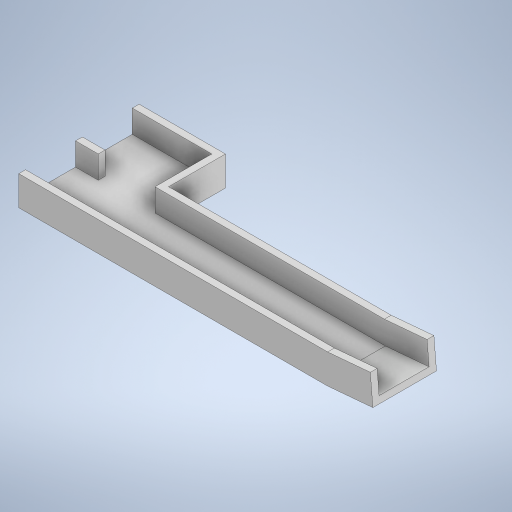
# Autodesk Inventor part: Trilho 5 min
Saved by Autodesk Inventor 2024 (Build 280153020, 153B)
## iProperties
Created: 2023-05-22
Part Number: Trilho 5 min
Material: Genérico
Document SubType Name: Modeling
Designer: jpjoa
Density: 1 g/cm^3
Appearance: Padrão
Author: jpjoa
Autodesk Inventor part; units mm, degrees
ref_plane "YZ Plane" through (0, 0, 0) normal (1, 0, 0) x (0, 1, 0)
ref_plane "XZ Plane" through (0, 0, 0) normal (0, 1, 0) x (-1, 0, 0)
sketch "Esboço1" plane through (0, 0, 0) normal (0, 1, 0) x (-1, 0, 0)
  line L0 (-133, -3) -> (0, -3)
  line L1 (0, -25) -> (-98, -25)
  line L2 (-133, 0) -> (-133, -28)
  line L3 (-133, -28) -> (-123, -28)
  line L4 (-95, -28) -> (0, -28)
  line L5 (0, -28) -> (0, 0)
  line L6 (0, 0) -> (-133, 0)
  line L7 (-95, -28) -> (-95, -53)
  line L8 (-95, -53) -> (-133, -53)
  line L9 (-133, -53) -> (-133, -50)
  line L10 (-133, -50) -> (-98, -50)
  line L11 (-98, -50) -> (-98, -25)
  arc A0 (-123, -50) -> (-98, -25) centre (-123, -25) ccw
  arc A1 (-123, -28) -> (-120, -25) centre (-123, -25) ccw
  line L12 (-133, -25) -> (-120, -25)
  line L13 (0, 0) -> (3, 0)
  line L14 (3, 0) -> (3, -28)
  line L15 (3, -28) -> (0, -28)
  line L16 (-123, -28) -> (-123, -25)
  line L17 (-133, -50) -> (-133, -28)
  line L18 (0, -3) -> (3, -3)
  line L19 (0, -25) -> (3, -25)
  line L20 (-133, -3) -> (-266, -3)
  line L21 (-266, -25) -> (-168, -25)
  line L22 (-133, -28) -> (-143, -28)
  line L23 (-171, -28) -> (-266, -28)
  line L24 (-266, -28) -> (-266, 0)
  line L25 (-266, 0) -> (-133, 0)
  line L26 (-171, -28) -> (-171, -53)
  line L27 (-171, -53) -> (-133, -53)
  line L28 (-133, -50) -> (-168, -50)
  line L29 (-168, -50) -> (-168, -25)
  arc A2 (-168, -25) -> (-143, -50) centre (-143, -25) ccw
  arc A3 (-146, -25) -> (-143, -28) centre (-143, -25) ccw
  line L30 (-133, -25) -> (-146, -25)
  line L31 (-266, 0) -> (-269, 0)
  line L32 (-269, 0) -> (-269, -28)
  line L33 (-269, -28) -> (-266, -28)
  line L34 (-143, -28) -> (-143, -25)
  line L35 (-266, -3) -> (-269, -3)
  line L36 (-266, -25) -> (-269, -25)
  point P0 (-133, -14)
  point P1 (-133, -51.5)
  point P2 (-83, -28)
  dimension "d7" = 22
  dimension "d9" = 3
  dimension "d10" = 3
  dimension "d13" = 3
  dimension "d14" = 3
  dimension "d16" = 22
  dimension "d20" = 22
  dimension "d21" = 120
  dimension "d29" = 3
  dimension "d31" = 10
  constraints: 74 end point, 17 symmetric about line, 12 point on line, 10 perpendicular, 8 point on circle, 4 centre point, 4 horizontal, 3 horizontal alignment, 2 coincident, 2 midpoint, 2 vertical, 2 vertical alignment, 1 collinear, 2 other
  measures "d7" distance between parallel lines of L0 L1
  measures "d9" distance between parallel lines of L1 L4
  measures "d10" distance between parallel lines of L6 L0
  measures "d13" distance between parallel lines of L11 L7
  measures "d14" distance between parallel lines of L10 L8
  measures "d16" distance between parallel lines of L10 L4
  measures "d20" radial gap between concentric circles of A0 A1
  measures "d21" distance from line of L5 L12.end
  measures "d29" distance between parallel lines of L14 L5
  measures "d31" distance of L9.end A0.start
extrude "Extrusão1" add sketch "Esboço1" against normal blind 3 contours L20 L24 L25 L2 | L2 L30 A3 L22 L17 L28 A2 L21 L24 L20 | L2 L22 L34 L30 | L35 L32 L31 L24 | L24 L36 L32 L35 | L34 A3 L30 | L21 L29 L28 L9 L27 L26 L23 L24 | L24 L33 L32 L36 | A2 L28 L29
extrude "Extrusão2" add sketch "Esboço1" along normal blind 10 contours L20 L24 L25 L2 | L2 L22 L34 L30 | L35 L32 L31 L24 | L21 L29 L28 L9 L27 L26 L23 L24 | L24 L33 L32 L36
sketch "Esboço2" plane through (133, -3, 0) normal (0, 0, 1) x (1, 0, 0)
  line L0 (0, 13) -> (136, 13) projected
  line L1 (136, 0) -> (0, 0) projected
  line L2 (136, 0) -> (155.9239, 1.7431)
  line L3 (136, 0) -> (156, 0) construction
  line L4 (155.9239, 1.7431) -> (154.7952, 14.6444)
  line L5 (154.7952, 14.6444) -> (136, 13)
  line L6 (136, 0) -> (136, 13) projected
  line L7 (136, 0) -> (136, 13)
  dimension "d32" = 20
  dimension "d33" = 5
  constraints: 10 end point, 2 perpendicular, 1 equal length, 1 horizontal, 1 vertical
  measures "d32" distance of L1.start L2.end
  measures "d33" angle of L3 L2
extrude "Extrusão4" add sketch "Esboço2" against normal up to surface (28 mm away)
ref_plane "Plano de trabalho1" through (171, -3, -14) normal (0, 0, -1) x (-1, 0, 0)
sketch "Esboço3" plane through (171, -3, -14) normal (0, 0, -1) x (-1, 0, 0)
  line L0 (-116.7952, 14.6444) -> (-98, 13) projected
  line L1 (3, 13) -> (-98, 13) projected
  line L2 (-98, 0) -> (-117.9239, 1.7431) projected
  line L3 (-117.6667, 4.6824) -> (-98.4366, 3)
  line L4 (-98.4366, 3) -> (-98, 3)
  line L5 (-117.9239, 1.7431) -> (-116.7952, 14.6444) projected
  line L6 (-117.6667, 4.6824) -> (-116.7952, 14.6444)
  line L7 (-116.7952, 14.6444) -> (-98, 13)
  line L8 (-98, 13) -> (-98, 3)
  dimension "d36" = 10
  constraints: 11 end point, 2 collinear, 1 vertical, 1 other
  measures "d36" distance between parallel lines of L0 L3
extrude "Extrusão5" cut sketch "Esboço3" along normal mid plane 22
equation "\"d9\" = mdf"
equation "\"d10\" = mdf"
equation "\"d13\" = mdf"
equation "\"d14\" = mdf"
equation "\"mdf\" = 3"
equation "\"margem\" = 1"
